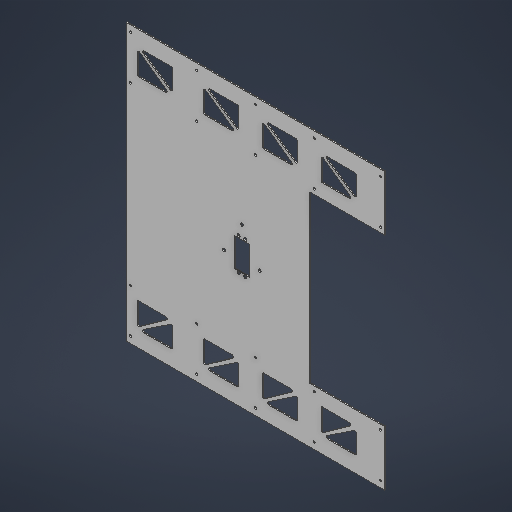
# Autodesk Inventor part: ВЕРХ 25-26
Saved by Autodesk Inventor 2026.2 (Build 302298000, 298)
## iProperties
Created: 2025-09-28
Part Number: ВЕРХ 25-26
Material: Типовые
Document SubType Name: Modeling
Designer: GameHD
Density: 1 g/cm^3
Appearance: По умолчанию
Author: GameHD
Autodesk Inventor part; units mm, degrees
(part 1 of 2)
ref_plane "YZ Plane" through (0, 0, 0) normal (1, 0, 0) x (0, 1, 0)
ref_plane "XZ Plane" through (0, 0, 0) normal (0, 1, 0) x (-1, 0, 0)
ref_plane "XY Plane" through (0, 0, 0) normal (0, 0, 1) x (1, 0, 0)
sketch "Эскиз1" plane through (0, 0, 0) normal (0, 0, 1) x (1, 0, 0)
  line L0 (0, 0) -> (380, 0)
  line L1 (380, 0) -> (380, 406)
  line L2 (380, 406) -> (0, 406)
  line L3 (0, 406) -> (0, 0)
  circle A0 centre (189.9999, 9.5) radius 1.625
  circle A1 centre (276.4236, 9.5) radius 1.625
  circle A2 centre (103.5763, 9.5) radius 1.625
  circle A3 centre (373.8998, 9.5) radius 1.625
  circle A4 centre (6.1, 9.5) radius 1.625
  line L4 (0, -31.725) -> (0, 41.275)
  line L5 (0, 203) -> (417.5125, 203)
  circle A5 centre (189.9999, 396.5) radius 1.625
  circle A6 centre (276.4236, 396.5) radius 1.625
  circle A7 centre (373.8998, 396.5) radius 1.625
  circle A8 centre (103.5763, 396.5) radius 1.625
  circle A9 centre (6.1, 396.5) radius 1.625
  circle A10 centre (189.9999, 73.9532) radius 1.625
  circle A11 centre (276.4236, 73.9532) radius 1.625
  circle A12 centre (373.8998, 73.9532) radius 1.625
  circle A13 centre (103.5763, 73.9532) radius 1.625
  circle A14 centre (6.1, 73.9532) radius 1.625
  circle A15 centre (189.9999, 332.0468) radius 1.625
  circle A16 centre (103.5763, 332.0468) radius 1.625
  circle A17 centre (373.8998, 332.0468) radius 1.625
  circle A18 centre (6.1, 332.0468) radius 1.625
  circle A19 centre (276.4236, 332.0468) radius 1.625
  line L6 (380, 203) -> (280, 203)
  line L7 (280, 203) -> (280, 81)
  line L8 (280, 81) -> (380, 81)
  line L9 (380, 81) -> (380, 203)
  line L10 (280, 203) -> (280, 325)
  line L11 (280, 325) -> (380, 325)
  circle A20 centre (6.1, 401.6) radius 1.625 projected
  arc A21 (257.5001, 384.25) -> (253.5001, 388.25) centre (253.5001, 384.25) ccw projected
  line L12 (253.5001, 388.25) -> (186.5001, 388.25) projected
  arc A22 (186.5001, 388.25) -> (182.5001, 384.25) centre (186.5001, 384.25) ccw projected
  line L13 (182.5001, 384.25) -> (182.5001, 342.25) projected
  arc A23 (182.5001, 342.25) -> (186.5001, 338.25) centre (186.5001, 342.25) ccw projected
  line L14 (186.5001, 338.25) -> (253.5001, 338.25) projected
  arc A24 (253.5001, 338.25) -> (257.5001, 342.25) centre (253.5001, 342.25) ccw projected
  line L15 (257.5001, 342.25) -> (257.5001, 384.25) projected
  line L16 (253.5001, 67.75) -> (186.5001, 67.75) projected
  arc A25 (186.5001, 67.75) -> (182.5001, 63.75) centre (186.5001, 63.75) ccw projected
  line L17 (182.5001, 63.75) -> (182.5001, 21.75) projected
  arc A26 (182.5001, 21.75) -> (186.5001, 17.75) centre (186.5001, 21.75) ccw projected
  line L18 (186.5001, 17.75) -> (253.5001, 17.75) projected
  arc A27 (253.5001, 17.75) -> (257.5001, 21.75) centre (253.5001, 21.75) ccw projected
  line L19 (257.5001, 21.75) -> (257.5001, 63.75) projected
  arc A28 (257.5001, 63.75) -> (253.5001, 67.75) centre (253.5001, 63.75) ccw projected
  arc A29 (148.6202, 331.9218) -> (145.3798, 331.9218) centre (147, 332.0468) ccw projected
  arc A30 (145.3798, 331.9218) -> (148.6202, 331.9218) centre (147, 331.7968) ccw projected
  arc A31 (371.3798, 314.6718) -> (374.6202, 314.6718) centre (373, 314.5468) ccw projected
  arc A32 (374.6202, 314.6718) -> (371.3798, 314.6718) centre (373, 314.7968) ccw projected
  arc A33 (231.3798, 74.0782) -> (234.6202, 74.0782) centre (233, 73.9532) ccw projected
  arc A34 (234.6202, 74.0782) -> (231.3798, 74.0782) centre (233, 74.2032) ccw projected
  arc A35 (5.38, 74.0782) -> (8.6204, 74.0782) centre (7.0002, 73.9532) ccw projected
  arc A36 (8.6204, 74.0782) -> (5.38, 74.0782) centre (7.0002, 74.2032) ccw projected
  arc A37 (148.6202, 91.3282) -> (145.3798, 91.3282) centre (147, 91.4532) ccw projected
  arc A38 (145.3798, 91.3282) -> (148.6202, 91.3282) centre (147, 91.2032) ccw projected
  arc A39 (374.6202, 91.3282) -> (371.3798, 91.3282) centre (373, 91.4532) ccw projected
  arc A40 (371.3798, 91.3282) -> (374.6202, 91.3282) centre (373, 91.2032) ccw projected
  arc A41 (231.3798, 314.6718) -> (234.6202, 314.6718) centre (233, 314.5468) ccw projected
  arc A42 (234.6202, 314.6718) -> (231.3798, 314.6718) centre (233, 314.7968) ccw projected
  arc A43 (5.38, 314.6718) -> (8.6204, 314.6718) centre (7.0002, 314.5468) ccw projected
  arc A44 (8.6204, 314.6718) -> (5.38, 314.6718) centre (7.0002, 314.7968) ccw projected
  arc A45 (145.3798, 314.6718) -> (148.6202, 314.6718) centre (147, 314.5468) ccw projected
  arc A46 (148.6202, 314.6718) -> (145.3798, 314.6718) centre (147, 314.7968) ccw projected
  arc A47 (374.6202, 331.9218) -> (371.3798, 331.9218) centre (373, 332.0468) ccw projected
  arc A48 (371.3798, 331.9218) -> (374.6202, 331.9218) centre (373, 331.7968) ccw projected
  arc A49 (234.6202, 91.3282) -> (231.3798, 91.3282) centre (233, 91.4532) ccw projected
  arc A50 (231.3798, 91.3282) -> (234.6202, 91.3282) centre (233, 91.2032) ccw projected
  arc A51 (8.6204, 91.3282) -> (5.38, 91.3282) centre (7.0002, 91.4532) ccw projected
  arc A52 (5.38, 91.3282) -> (8.6204, 91.3282) centre (7.0002, 91.2032) ccw projected
  arc A53 (145.3798, 74.0782) -> (148.6202, 74.0782) centre (147, 73.9532) ccw projected
  arc A54 (148.6202, 74.0782) -> (145.3798, 74.0782) centre (147, 74.2032) ccw projected
  arc A55 (371.3798, 74.0782) -> (374.6202, 74.0782) centre (373, 73.9532) ccw projected
  arc A56 (374.6202, 74.0782) -> (371.3798, 74.0782) centre (373, 74.2032) ccw projected
  arc A57 (234.6202, 331.9218) -> (231.3798, 331.9218) centre (233, 332.0468) ccw projected
  arc A58 (231.3798, 331.9218) -> (234.6202, 331.9218) centre (233, 331.7968) ccw projected
  arc A59 (8.6204, 331.9218) -> (5.38, 331.9218) centre (7.0002, 332.0468) ccw projected
  arc A60 (5.38, 331.9218) -> (8.6204, 331.9218) centre (7.0002, 331.7968) ccw projected
  circle A61 centre (373.9, 401.6) radius 1.625 projected
  circle A62 centre (374, 4.4) radius 1.625 projected
  circle A63 centre (6.1, 401.6) radius 1.625 projected
  circle A64 centre (6.1, 4.4) radius 1.625 projected
  circle A65 centre (190.0848, 396.5) radius 1.625 projected
  circle A66 centre (190.0848, 9.5) radius 1.625 projected
  circle A67 centre (233, 396.5) radius 1.625 projected
  circle A68 centre (233, 9.5) radius 1.625 projected
  circle A69 centre (134.0059, 201.175) radius 1.85 projected
  arc A70 (197.7028, 203) -> (198.309, 203) centre (198.0059, 201.175) ccw projected
  line L20 (198.309, 203) -> (197.7028, 203) projected
  circle A71 centre (134.0059, 142.375) radius 2 projected
  circle A72 centre (317.9941, 235.25) radius 2.1 projected
  circle A73 centre (62.0059, 170.75) radius 2.1 projected
  circle A74 centre (123.0059, 170.75) radius 2.1 projected
  circle A75 centre (317.9941, 170.75) radius 2.1 projected
  circle A76 centre (256.9941, 235.25) radius 2.1 projected
  circle A77 centre (62.0059, 235.25) radius 2.1 projected
  circle A78 centre (123.0059, 235.25) radius 2.1 projected
  circle A79 centre (256.9941, 170.75) radius 2.1 projected
  line L21 (49, 183) -> (13, 183) projected
  arc A80 (13, 183) -> (10, 180) centre (13, 180) ccw projected
  line L22 (10, 180) -> (10, 114) projected
  arc A81 (10, 114) -> (13, 111) centre (13, 114) ccw projected
  line L23 (13, 111) -> (49, 111) projected
  arc A82 (49, 111) -> (52, 114) centre (49, 114) ccw projected
  line L24 (52, 114) -> (52, 180) projected
  arc A83 (52, 180) -> (49, 183) centre (49, 180) ccw projected
  circle A84 centre (170.0002, 337.1128) radius 2.1 projected
  circle A85 centre (61.343, 305) radius 2.1 projected
  circle A86 centre (170.0002, 68.8872) radius 2.1 projected
  circle A87 centre (61.343, 191.9908) radius 2.1 projected
  circle A88 centre (65, 153.25) radius 2.1 projected
  circle A89 centre (65, 121) radius 2.1 projected
  arc A90 (32.152, 58) -> (34.152, 60) centre (32.152, 60) ccw projected
  line L25 (32.152, 58) -> (8, 58) projected
  arc A91 (8, 58) -> (5, 55) centre (8, 55) ccw projected
  line L26 (5, 55) -> (5, 11) projected
  arc A92 (5, 11) -> (8, 8) centre (8, 11) ccw projected
  line L27 (8, 8) -> (165, 8) projected
  arc A93 (165, 8) -> (168, 11) centre (165, 11) ccw projected
  line L28 (168, 11) -> (168, 55) projected
  arc A94 (168, 55) -> (165, 58) centre (165, 55) ccw projected
  line L29 (165, 58) -> (116.152, 58) projected
  arc A95 (114.152, 60) -> (116.152, 58) centre (116.152, 60) ccw projected
  line L30 (114.152, 60) -> (114.152, 72) projected
  arc A96 (114.152, 72) -> (112.152, 74) centre (112.152, 72) ccw projected
  line L31 (112.152, 74) -> (36.152, 74) projected
  arc A97 (36.152, 74) -> (34.152, 72) centre (36.152, 72) ccw projected
  line L32 (34.152, 72) -> (34.152, 60) projected
  arc A98 (345.848, 60) -> (347.848, 58) centre (347.848, 60) ccw projected
  line L33 (345.848, 60) -> (345.848, 72) projected
  arc A99 (345.848, 72) -> (343.848, 74) centre (343.848, 72) ccw projected
  line L34 (343.848, 74) -> (267.848, 74) projected
  arc A100 (267.848, 74) -> (265.848, 72) centre (267.848, 72) ccw projected
  line L35 (265.848, 72) -> (265.848, 10) projected
  arc A101 (265.848, 10) -> (267.848, 8) centre (267.848, 10) ccw projected
  line L36 (267.848, 8) -> (372, 8) projected
  arc A102 (372, 8) -> (375, 11) centre (372, 11) ccw projected
  line L37 (375, 11) -> (375, 55) projected
  arc A103 (375, 55) -> (372, 58) centre (372, 55) ccw projected
  line L38 (372, 58) -> (347.848, 58) projected
  arc A104 (347.848, 348) -> (345.848, 346) centre (347.848, 346) ccw projected
  line L39 (347.848, 348) -> (372, 348) projected
  arc A105 (372, 348) -> (375, 351) centre (372, 351) ccw projected
  line L40 (375, 351) -> (375, 395) projected
  arc A106 (375, 395) -> (372, 398) centre (372, 395) ccw projected
  line L41 (372, 398) -> (267.848, 398) projected
  arc A107 (267.848, 398) -> (265.848, 396) centre (267.848, 396) ccw projected
  line L42 (265.848, 396) -> (265.848, 334) projected
  arc A108 (265.848, 334) -> (267.848, 332) centre (267.848, 334) ccw projected
  line L43 (267.848, 332) -> (343.848, 332) projected
  arc A109 (343.848, 332) -> (345.848, 334) centre (343.848, 334) ccw projected
  line L44 (345.848, 334) -> (345.848, 346) projected
  arc A110 (34.152, 346) -> (32.152, 348) centre (32.152, 346) ccw projected
  line L45 (34.152, 346) -> (34.152, 334) projected
  arc A111 (34.152, 334) -> (36.152, 332) centre (36.152, 334) ccw projected
  line L46 (36.152, 332) -> (112.152, 332) projected
  arc A112 (112.152, 332) -> (114.152, 334) centre (112.152, 334) ccw projected
  line L47 (114.152, 334) -> (114.152, 346) projected
  arc A113 (116.152, 348) -> (114.152, 346) centre (116.152, 346) ccw projected
  line L48 (116.152, 348) -> (165, 348) projected
  arc A114 (165, 348) -> (168, 351) centre (165, 351) ccw projected
  line L49 (168, 351) -> (168, 395) projected
  arc A115 (168, 395) -> (165, 398) centre (165, 395) ccw projected
  line L50 (165, 398) -> (8, 398) projected
  arc A116 (8, 398) -> (5, 395) centre (8, 395) ccw projected
  line L51 (5, 395) -> (5, 351) projected
  arc A117 (5, 351) -> (8, 348) centre (8, 351) ccw projected
  line L52 (8, 348) -> (32.152, 348) projected
  line L53 (176.1539, 208.9063) -> (141.4028, 224.6949) projected
  arc A118 (141.4028, 224.6949) -> (137.8279, 220.0788) centre (140.1619, 221.9636) ccw projected
  line L54 (137.8279, 220.0788) -> (150.5778, 204.2902) projected
  arc A119 (150.5778, 204.2902) -> (152.9118, 203.175) centre (152.9118, 206.175) ccw projected
  line L55 (152.9118, 203.175) -> (174.913, 203.175) projected
  arc A120 (174.913, 203.175) -> (176.1539, 208.9063) centre (174.913, 206.175) ccw projected
  line L56 (164.9717, 173.5408) -> (165.9394, 174.4298) projected
  arc A121 (165.9394, 174.4298) -> (166.2437, 178.5238) centre (163.9097, 176.639) ccw projected
  line L57 (166.2437, 178.5238) -> (150.4677, 198.0598) projected
  arc A122 (150.4677, 198.0598) -> (148.1337, 199.175) centre (148.1337, 196.175) ccw projected
  line L58 (148.1337, 199.175) -> (145.4623, 199.175) projected
  arc A123 (145.4623, 199.175) -> (142.7128, 197.375) centre (145.4623, 196.175) ccw projected
  arc A124 (137.8059, 192.4681) -> (142.7128, 197.375) centre (134.0059, 201.175) ccw projected
  arc A125 (137.8059, 192.4681) -> (136.0059, 189.7186) centre (139.0059, 189.7186) ccw projected
  line L59 (136.0059, 189.7186) -> (136.0059, 175.75) projected
  arc A126 (136.0059, 175.75) -> (139.0059, 172.75) centre (139.0059, 175.75) ccw projected
  line L60 (139.0059, 172.75) -> (162.942, 172.75) projected
  arc A127 (162.942, 172.75) -> (164.9717, 173.5408) centre (162.942, 175.75) ccw projected
  line L61 (190.9762, 192.0005) -> (175.6931, 177.9592) projected
  arc A128 (175.6931, 177.9592) -> (177.7227, 172.75) centre (177.7227, 175.75) ccw projected
  line L62 (177.7227, 172.75) -> (193.0059, 172.75) projected
  arc A129 (193.0059, 172.75) -> (196.0059, 175.75) centre (193.0059, 175.75) ccw projected
  line L63 (196.0059, 175.75) -> (196.0059, 189.7914) projected
  arc A130 (196.0059, 189.7914) -> (190.9762, 192.0005) centre (193.0059, 189.7914) ccw projected
  line L64 (75.0034, 126.1924) -> (112.8628, 137.9196) projected
  arc A131 (112.8628, 137.9196) -> (112.4422, 143.7487) centre (111.9752, 140.7852) ccw projected
  line L65 (112.4422, 143.7487) -> (74.5828, 149.7151) projected
  arc A132 (74.5828, 149.7151) -> (71.1158, 146.7517) centre (74.1158, 146.7517) ccw projected
  line L66 (71.1158, 146.7517) -> (71.1158, 129.058) projected
  arc A133 (71.1158, 129.058) -> (75.0034, 126.1924) centre (74.1158, 129.058) ccw projected
  line L67 (273.1271, 237.25) -> (305.3345, 237.25) projected
  arc A134 (305.3345, 237.25) -> (307.3845, 242.4403) centre (305.3345, 240.25) ccw projected
  line L68 (307.3845, 242.4403) -> (293.7654, 255.1866) projected
  arc A135 (293.7654, 255.1866) -> (290.0188, 255.4704) centre (291.7154, 252.9963) ccw projected
  line L69 (290.0188, 255.4704) -> (271.4305, 242.7242) projected
  arc A136 (271.4305, 242.7242) -> (273.1271, 237.25) centre (273.1271, 240.25) ccw projected
  line L70 (237.7677, 178.4162) -> (207.2709, 194.1459) projected
  arc A137 (207.2709, 194.1459) -> (204.0022, 193.8065) centre (205.8957, 191.4797) ccw projected
  arc A138 (201.8059, 192.4681) -> (204.0022, 193.8065) centre (198.0059, 201.175) ccw projected
  arc A139 (201.8059, 192.4681) -> (200.0059, 189.7186) centre (203.0059, 189.7186) ccw projected
  line L71 (200.0059, 189.7186) -> (200.0059, 175.75) projected
  arc A140 (200.0059, 175.75) -> (203.0059, 172.75) centre (203.0059, 175.75) ccw projected
  line L72 (203.0059, 172.75) -> (236.3925, 172.75) projected
  arc A141 (236.3925, 172.75) -> (237.7677, 178.4162) centre (236.3925, 175.75) ccw projected
  line L73 (171.7502, 299.3659) -> (188.242, 287.4391) projected
  arc A142 (188.242, 287.4391) -> (191.758, 287.4391) centre (190, 289.8701) ccw projected
  line L74 (191.758, 287.4391) -> (215.7595, 304.7968) projected
  line L75 (215.7595, 304.7968) -> (173.5082, 304.7968) projected
  arc A143 (173.5082, 304.7968) -> (171.7502, 299.3659) centre (173.5082, 301.7968) ccw projected
  line L76 (265.3115, 243.3784) -> (285.9348, 257.5201) projected
  arc A144 (285.9348, 257.5201) -> (286.2882, 262.1846) centre (284.2382, 259.9942) ccw projected
  line L77 (286.2882, 262.1846) -> (245.2049, 300.6348) projected
  arc A145 (245.2049, 300.6348) -> (240.2828, 297.5781) centre (243.1549, 298.4444) ccw projected
  line L78 (240.2828, 297.5781) -> (255.6005, 246.7959) projected
  arc A146 (255.6005, 246.7959) -> (258.1178, 244.6833) centre (258.4726, 247.6622) ccw projected
  arc A147 (262.0259, 243.308) -> (258.1178, 244.6833) centre (256.9941, 235.25) ccw projected
  arc A148 (262.0259, 243.308) -> (265.3115, 243.3784) centre (263.6149, 245.8526) ccw projected
  arc A149 (72.6155, 242.4403) -> (74.6655, 237.25) centre (74.6655, 240.25) ccw projected
  line L79 (74.6655, 237.25) -> (111.9119, 237.25) projected
  arc A150 (111.9119, 237.25) -> (114.1595, 242.237) centre (111.9119, 240.25) ccw projected
  line L80 (114.1595, 242.237) -> (97.2953, 261.3129) projected
  arc A151 (97.2953, 261.3129) -> (92.9977, 261.5163) centre (95.0477, 259.3259) ccw projected
  line L81 (92.9977, 261.5163) -> (72.6155, 242.4403) projected
  line L82 (252.1574, 299.6064) -> (290.6344, 263.5955) projected
  arc A152 (290.6344, 263.5955) -> (294.3809, 263.3117) centre (292.6843, 265.7859) ccw projected
  line L83 (294.3809, 263.3117) -> (316.6907, 278.6098) projected
  arc A153 (316.6907, 278.6098) -> (317.9941, 281.084) centre (314.9941, 281.084) ccw projected
  line L84 (317.9941, 281.084) -> (317.9941, 301.7968) projected
  arc A154 (317.9941, 301.7968) -> (314.9941, 304.7968) centre (314.9941, 301.7968) ccw projected
  line L85 (314.9941, 304.7968) -> (254.2074, 304.7968) projected
  arc A155 (254.2074, 304.7968) -> (252.1574, 299.6064) centre (254.2074, 301.7968) ccw projected
  line L86 (196.7743, 281.2686) -> (212.8517, 269.6416) projected
  arc A156 (212.8517, 269.6416) -> (217.4768, 271.1895) centre (214.6097, 272.0726) ccw projected
  line L87 (217.4768, 271.1895) -> (226.6315, 300.9138) projected
  arc A157 (226.6315, 300.9138) -> (223.7644, 304.7968) centre (223.7644, 301.7968) ccw projected
  line L88 (223.7644, 304.7968) -> (223.5564, 304.7968) projected
  arc A158 (223.5564, 304.7968) -> (221.7984, 304.2277) centre (223.5564, 301.7968) ccw projected
  line L89 (221.7984, 304.2277) -> (196.7743, 286.1305) projected
  arc A159 (196.7743, 286.1305) -> (196.7743, 281.2686) centre (198.5323, 283.6996) ccw projected
  line L90 (209.1045, 197.7009) -> (247.729, 177.7791) projected
  arc A160 (247.729, 177.7791) -> (250.9978, 178.1185) centre (249.1042, 180.4453) ccw projected
  arc A161 (253.1941, 179.4569) -> (250.9978, 178.1185) centre (256.9941, 170.75) ccw projected
  arc A162 (253.1941, 179.4569) -> (254.9941, 182.2064) centre (251.9941, 182.2064) ccw projected
  line L91 (254.9941, 182.2064) -> (254.9941, 223.7936) projected
  arc A163 (254.9941, 223.7936) -> (253.1941, 226.5431) centre (251.9941, 223.7936) ccw projected
  arc A164 (251.3555, 227.6044) -> (253.1941, 226.5431) centre (256.9941, 235.25) ccw projected
  arc A165 (251.3555, 227.6044) -> (248.0743, 227.7877) centre (249.5749, 225.1899) ccw projected
  line L92 (248.0743, 227.7877) -> (208.9265, 205.1737) projected
  arc A166 (208.9265, 205.1737) -> (207.446, 202.2397) centre (210.4271, 202.576) ccw projected
  arc A167 (207.486, 200.561) -> (207.446, 202.2397) centre (198.0059, 201.175) ccw projected
  arc A168 (207.486, 200.561) -> (209.1045, 197.7009) centre (210.4797, 200.3671) ccw projected
  line L93 (290.6344, 142.4045) -> (250.0205, 104.3936) projected
  arc A169 (250.0205, 104.3936) -> (252.0705, 99.2032) centre (252.0705, 102.2032) ccw projected
  line L94 (252.0705, 99.2032) -> (314.9941, 99.2032) projected
  arc A170 (314.9941, 99.2032) -> (317.9941, 102.2032) centre (314.9941, 102.2032) ccw projected
  line L95 (317.9941, 102.2032) -> (317.9941, 124.916) projected
  arc A171 (317.9941, 124.916) -> (316.6907, 127.3902) centre (314.9941, 124.916) ccw projected
  line L96 (316.6907, 127.3902) -> (294.3809, 142.6883) projected
  arc A172 (294.3809, 142.6883) -> (290.6344, 142.4045) centre (292.6843, 140.2141) ccw projected
  line L97 (258.9941, 222.6864) -> (258.9941, 183.3136) projected
  arc A173 (258.9941, 183.3136) -> (264.1737, 181.2523) centre (261.9941, 183.3136) ccw projected
  line L98 (264.1737, 181.2523) -> (282.7918, 200.9386) projected
  arc A174 (282.7918, 200.9386) -> (282.7918, 205.0614) centre (280.6122, 203) ccw projected
  line L99 (282.7918, 205.0614) -> (264.1737, 224.7477) projected
  arc A175 (264.1737, 224.7477) -> (258.9941, 222.6864) centre (261.9941, 222.6864) ccw projected
  line L100 (73.6488, 153.9117) -> (89.4125, 151.4274) projected
  arc A176 (89.4125, 151.4274) -> (90.9794, 157.1819) centre (89.8795, 154.3908) ccw projected
  line L101 (90.9794, 157.1819) -> (75.2157, 163.3943) projected
  arc A177 (75.2157, 163.3943) -> (71.1158, 160.6033) centre (74.1158, 160.6033) ccw projected
  line L102 (71.1158, 160.6033) -> (71.1158, 156.8751) projected
  arc A178 (71.1158, 156.8751) -> (73.6488, 153.9117) centre (74.1158, 156.8751) ccw projected
  line L103 (136.0059, 165.75) -> (136.0059, 153.7586) projected
  arc A179 (136.0059, 153.7586) -> (141.0355, 151.5495) centre (139.0059, 153.7586) ccw projected
  line L104 (141.0355, 151.5495) -> (154.0874, 163.5408) projected
  arc A180 (154.0874, 163.5408) -> (152.0577, 168.75) centre (152.0577, 165.75) ccw projected
  line L105 (152.0577, 168.75) -> (139.0059, 168.75) projected
  arc A181 (139.0059, 168.75) -> (136.0059, 165.75) centre (139.0059, 165.75) ccw projected
  line L106 (187.6976, 229.0214) -> (194.3962, 214.0995) projected
  arc A182 (194.3962, 214.0995) -> (200.0002, 214.4451) centre (197.1331, 215.3281) ccw projected
  line L107 (200.0002, 214.4451) -> (204.5959, 229.367) projected
  arc A183 (204.5959, 229.367) -> (201.7288, 233.25) centre (201.7288, 230.25) ccw projected
  line L108 (201.7288, 233.25) -> (190.4345, 233.25) projected
  arc A184 (190.4345, 233.25) -> (187.6976, 229.0214) centre (190.4345, 230.25) ccw projected
  line L109 (96.148, 187.9448) -> (84.8346, 202.5382) projected
  arc A185 (84.8346, 202.5382) -> (80.7407, 203.156) centre (82.4637, 200.7001) ccw projected
  line L110 (80.7407, 203.156) -> (72.3928, 197.2996) projected
  arc A186 (72.3928, 197.2996) -> (71.1158, 194.8437) centre (74.1158, 194.8437) ccw projected
  line L111 (71.1158, 194.8437) -> (71.1158, 192.8793) projected
  arc A187 (71.1158, 192.8793) -> (73.1387, 190.0429) centre (74.1158, 192.8793) ccw projected
  line L112 (73.1387, 190.0429) -> (92.8, 183.2703) projected
  arc A188 (92.8, 183.2703) -> (96.148, 187.9448) centre (93.777, 186.1067) ccw projected
  line L113 (158.6531, 194.2902) -> (168.9546, 181.5336) projected
  arc A189 (168.9546, 181.5336) -> (173.3182, 181.2092) centre (171.2886, 183.4184) ccw projected
  line L114 (173.3182, 181.2092) -> (187.203, 193.9658) projected
  arc A190 (187.203, 193.9658) -> (185.1733, 199.175) centre (185.1733, 196.175) ccw projected
  line L115 (185.1733, 199.175) -> (160.9871, 199.175) projected
  arc A191 (160.9871, 199.175) -> (158.6531, 194.2902) centre (160.9871, 196.175) ccw projected
  line L116 (88.7233, 213.6423) -> (108.8956, 227.7941) projected
  arc A192 (108.8956, 227.7941) -> (107.1727, 233.25) centre (107.1727, 230.25) ccw projected
  line L117 (107.1727, 233.25) -> (74.1158, 233.25) projected
  arc A193 (74.1158, 233.25) -> (71.1158, 230.25) centre (74.1158, 230.25) ccw projected
  line L118 (71.1158, 230.25) -> (71.1158, 229.722) projected
  arc A194 (71.1158, 229.722) -> (71.9361, 227.6607) centre (74.1158, 229.722) ccw projected
  line L119 (71.9361, 227.6607) -> (84.8207, 214.0368) projected
  arc A195 (84.8207, 214.0368) -> (88.7233, 213.6423) centre (87.0003, 216.0982) ccw projected
  line L120 (138.452, 237.25) -> (174.984, 237.25) projected
  arc A196 (174.984, 237.25) -> (177.7209, 241.4786) centre (174.984, 240.25) ccw projected
  line L121 (177.7209, 241.4786) -> (168.7676, 261.4233) projected
  arc A197 (168.7676, 261.4233) -> (164.2727, 262.6256) centre (166.0307, 260.1947) ccw projected
  line L122 (164.2727, 262.6256) -> (136.694, 242.6809) projected
  arc A198 (136.694, 242.6809) -> (138.452, 237.25) centre (138.452, 240.25) ccw projected
  line L123 (183.2224, 163.8652) -> (190.6719, 154.6403) projected
  arc A199 (190.6719, 154.6403) -> (196.0059, 156.5251) centre (193.0059, 156.5251) ccw projected
  line L124 (196.0059, 156.5251) -> (196.0059, 165.75) projected
  arc A200 (196.0059, 165.75) -> (193.0059, 168.75) centre (193.0059, 165.75) ccw projected
  line L125 (193.0059, 168.75) -> (185.5564, 168.75) projected
  arc A201 (185.5564, 168.75) -> (183.2224, 163.8652) centre (185.5564, 165.75) ccw projected
  line L126 (104.4945, 108.7766) -> (129.3603, 99.741) projected
  arc A202 (129.3603, 99.741) -> (133.3849, 102.5606) centre (130.3849, 102.5606) ccw projected
  line L127 (133.3849, 102.5606) -> (133.3849, 108.9115) projected
  arc A203 (133.3849, 108.9115) -> (130.7069, 111.8942) centre (130.3849, 108.9115) ccw projected
  line L128 (130.7069, 111.8942) -> (105.8411, 114.5789) projected
  arc A204 (105.8411, 114.5789) -> (104.4945, 108.7766) centre (105.5191, 111.5962) ccw projected
  line L129 (266.425, 228.1886) -> (285.3145, 208.2154) projected
  arc A205 (285.3145, 208.2154) -> (289.6737, 208.2154) centre (287.4941, 210.2768) ccw projected
  line L130 (289.6737, 208.2154) -> (308.5632, 228.1886) projected
  arc A206 (308.5632, 228.1886) -> (306.3835, 233.25) centre (306.3835, 230.25) ccw projected
  line L131 (306.3835, 233.25) -> (268.6047, 233.25) projected
  arc A207 (268.6047, 233.25) -> (266.425, 228.1886) centre (268.6047, 230.25) ccw projected
  line L132 (76.1657, 251.2416) -> (90.4716, 264.6306) projected
  arc A208 (90.4716, 264.6306) -> (90.6693, 268.808) centre (88.4217, 266.821) ccw projected
  line L133 (90.6693, 268.808) -> (76.3634, 284.9901) projected
  arc A209 (76.3634, 284.9901) -> (71.1158, 283.0031) centre (74.1158, 283.0031) ccw projected
  line L134 (71.1158, 283.0031) -> (71.1158, 253.432) projected
  arc A210 (71.1158, 253.432) -> (76.1657, 251.2416) centre (74.1158, 253.432) ccw projected
  line L135 (133.824, 245.5418) -> (163.6065, 267.0802) projected
  arc A211 (163.6065, 267.0802) -> (164.5853, 270.7397) centre (161.8485, 269.5111) ccw projected
  line L136 (164.5853, 270.7397) -> (150.6579, 301.7648) projected
  arc A212 (150.6579, 301.7648) -> (145.0488, 301.4025) centre (147.921, 300.5362) ccw projected
  line L137 (145.0488, 301.4025) -> (129.1938, 248.8391) projected
  arc A213 (129.1938, 248.8391) -> (133.824, 245.5418) centre (132.066, 247.9727) ccw projected
  line L138 (71.8682, 296.1141) -> (93.4781, 271.6699) projected
  arc A214 (93.4781, 271.6699) -> (97.7757, 271.4666) centre (95.7258, 273.657) ccw projected
  line L139 (97.7757, 271.4666) -> (127.8426, 299.6064) projected
  arc A215 (127.8426, 299.6064) -> (125.7926, 304.7968) centre (125.7926, 301.7968) ccw projected
  line L140 (125.7926, 304.7968) -> (74.1158, 304.7968) projected
  arc A216 (74.1158, 304.7968) -> (71.1158, 301.7968) centre (74.1158, 301.7968) ccw projected
  line L141 (71.1158, 301.7968) -> (71.1158, 298.1011) projected
  arc A217 (71.1158, 298.1011) -> (71.8682, 296.1141) centre (74.1158, 298.1011) ccw projected
  line L142 (243.306, 242.6809) -> (221.8167, 258.2218) projected
  arc A218 (221.8167, 258.2218) -> (217.1916, 256.6739) centre (220.0587, 255.7909) ccw projected
  line L143 (217.1916, 256.6739) -> (212.4052, 241.133) projected
  arc A219 (212.4052, 241.133) -> (215.2723, 237.25) centre (215.2723, 240.25) ccw projected
  line L144 (215.2723, 237.25) -> (241.548, 237.25) projected
  arc A220 (241.548, 237.25) -> (243.306, 242.6809) centre (241.548, 240.25) ccw projected
  line L145 (207.6758, 239.367) -> (214.3683, 261.0966) projected
  arc A221 (214.3683, 261.0966) -> (213.2592, 264.4105) centre (211.5012, 261.9796) ccw projected
  line L146 (213.2592, 264.4105) -> (191.758, 279.96) projected
  arc A222 (191.758, 279.96) -> (188.242, 279.96) centre (190, 277.529) ccw projected
  line L147 (188.242, 279.96) -> (172.5476, 268.6099) projected
  arc A223 (172.5476, 268.6099) -> (171.5688, 264.9504) centre (174.3056, 266.179) ccw projected
  line L148 (171.5688, 264.9504) -> (183.2085, 239.0214) projected
  arc A224 (183.2085, 239.0214) -> (185.9454, 237.25) centre (185.9454, 240.25) ccw projected
  line L149 (185.9454, 237.25) -> (204.8087, 237.25) projected
  arc A225 (204.8087, 237.25) -> (207.6758, 239.367) centre (204.8087, 240.25) ccw projected
  line L150 (285.3145, 197.7846) -> (266.425, 177.8114) projected
  arc A226 (266.425, 177.8114) -> (268.6047, 172.75) centre (268.6047, 175.75) ccw projected
  line L151 (268.6047, 172.75) -> (306.3835, 172.75) projected
  arc A227 (306.3835, 172.75) -> (308.5632, 177.8114) centre (306.3835, 175.75) ccw projected
  line L152 (308.5632, 177.8114) -> (289.6737, 197.7846) projected
  arc A228 (289.6737, 197.7846) -> (285.3145, 197.7846) centre (287.4941, 195.7232) ccw projected
  line L153 (310.8145, 224.7477) -> (292.1964, 205.0614) projected
  arc A229 (292.1964, 205.0614) -> (292.1964, 200.9386) centre (294.376, 203) ccw projected
  line L154 (292.1964, 200.9386) -> (310.8145, 181.2523) projected
  arc A230 (310.8145, 181.2523) -> (315.9941, 183.3136) centre (312.9941, 183.3136) ccw projected
  line L155 (315.9941, 183.3136) -> (315.9941, 222.6864) projected
  arc A231 (315.9941, 222.6864) -> (310.8145, 224.7477) centre (312.9941, 222.6864) ccw projected
  line L156 (190.7609, 212.4306) -> (182.21, 231.4786) projected
  arc A232 (182.21, 231.4786) -> (179.4731, 233.25) centre (179.4731, 230.25) ccw projected
  line L157 (179.4731, 233.25) -> (146.0987, 233.25) projected
  arc A233 (146.0987, 233.25) -> (144.8578, 227.5187) centre (146.0987, 230.25) ccw projected
  line L158 (144.8578, 227.5187) -> (186.783, 208.4706) projected
  arc A234 (186.783, 208.4706) -> (190.7609, 212.4306) centre (188.024, 211.202) ccw projected
  line L159 (121.268, 155.5417) -> (111.9292, 167.5881) projected
  arc A235 (111.9292, 167.5881) -> (109.5582, 168.75) centre (109.5582, 165.75) ccw projected
  line L160 (109.5582, 168.75) -> (88.33, 168.75) projected
  arc A236 (88.33, 168.75) -> (87.2301, 162.9589) centre (88.33, 165.75) ccw projected
  line L161 (87.2301, 162.9589) -> (117.797, 150.9126) projected
  arc A237 (117.797, 150.9126) -> (121.268, 155.5417) centre (118.897, 153.7036) ccw projected
  line L162 (114.7758, 227.0332) -> (92.2222, 211.2108) projected
  arc A238 (92.2222, 211.2108) -> (91.7655, 206.6935) centre (93.9452, 208.7549) ccw projected
  line L163 (91.7655, 206.6935) -> (115.8263, 181.2523) projected
  arc A239 (115.8263, 181.2523) -> (121.0059, 183.3136) centre (118.0059, 183.3136) ccw projected
  line L164 (121.0059, 183.3136) -> (121.0059, 223.7936) projected
  arc A240 (121.0059, 223.7936) -> (119.2059, 226.5431) centre (118.0059, 223.7936) ccw projected
  arc A241 (118.0605, 227.1387) -> (119.2059, 226.5431) centre (123.0059, 235.25) ccw projected
  arc A242 (118.0605, 227.1387) -> (114.7758, 227.0332) centre (116.4988, 224.5773) ccw projected
  line L165 (285.9348, 148.4799) -> (283.4292, 150.1981) projected
  arc A243 (283.4292, 150.1981) -> (280.4301, 150.4264) centre (281.7326, 147.7239) ccw projected
  line L166 (280.4301, 150.4264) -> (242.0824, 131.9453) projected
  arc A244 (242.0824, 131.9453) -> (240.3849, 129.2428) centre (243.3849, 129.2428) ccw projected
  line L167 (240.3849, 129.2428) -> (240.3849, 107.7707) projected
  arc A245 (240.3849, 107.7707) -> (245.4348, 105.5804) centre (243.3849, 107.7707) ccw projected
  line L168 (245.4348, 105.5804) -> (286.2882, 143.8154) projected
  arc A246 (286.2882, 143.8154) -> (285.9348, 148.4799) centre (284.2382, 146.0058) ccw projected
  line L169 (139.3849, 123.75) -> (139.3849, 99.75) projected
  arc A247 (139.3849, 99.75) -> (142.3849, 96.75) centre (142.3849, 99.75) ccw projected
  line L170 (142.3849, 96.75) -> (231.3849, 96.75) projected
  arc A248 (231.3849, 96.75) -> (234.3849, 99.75) centre (231.3849, 99.75) ccw projected
  line L171 (234.3849, 99.75) -> (234.3849, 123.75) projected
  arc A249 (234.3849, 123.75) -> (231.3849, 126.75) centre (231.3849, 123.75) ccw projected
  line L172 (231.3849, 126.75) -> (142.3849, 126.75) projected
  arc A250 (142.3849, 126.75) -> (139.3849, 123.75) centre (142.3849, 123.75) ccw projected
  line L173 (134.7951, 300.6348) -> (100.3018, 268.3522) projected
  arc A251 (100.3018, 268.3522) -> (100.1042, 264.1749) centre (102.3518, 266.1619) ccw projected
  line L174 (100.1042, 264.1749) -> (116.9163, 245.1579) projected
  arc A252 (116.9163, 245.1579) -> (120.086, 244.2901) centre (119.1639, 247.1449) ccw projected
  arc A253 (121.8822, 244.6833) -> (120.086, 244.2901) centre (123.0059, 235.25) ccw projected
  arc A254 (121.8822, 244.6833) -> (124.3995, 246.7959) centre (121.5274, 247.6622) ccw projected
  line L175 (124.3995, 246.7959) -> (139.7172, 297.5781) projected
  arc A255 (139.7172, 297.5781) -> (134.7951, 300.6348) centre (136.8451, 298.4444) ccw projected
  arc A256 (133.3849, 129.2358) -> (133.1423, 131.1911) centre (125.3849, 129.2358) ccw projected
  arc A257 (133.1423, 131.1911) -> (131.1387, 133.318) centre (130.2332, 130.4579) ccw projected
  arc A258 (126.839, 136.1392) -> (131.1387, 133.318) centre (134.0059, 142.375) ccw projected
  arc A259 (126.839, 136.1392) -> (124.0903, 137.1304) centre (124.5758, 134.1699) ccw projected
  arc A260 (124.0903, 137.1304) -> (123.0178, 136.8776) centre (125.3849, 129.2358) ccw projected
  line L176 (123.0178, 136.8776) -> (88.6823, 126.242) projected
  arc A261 (88.6823, 126.242) -> (89.2479, 120.3937) centre (89.57, 123.3763) ccw projected
  line L177 (89.2479, 120.3937) -> (130.0629, 115.987) projected
  arc A262 (130.0629, 115.987) -> (133.3849, 118.9697) centre (130.3849, 118.9697) ccw projected
  line L178 (133.3849, 118.9697) -> (133.3849, 129.2358) projected
  line L179 (94.1155, 178.5864) -> (75.0928, 185.1391) projected
  arc A263 (75.0928, 185.1391) -> (71.1158, 182.3027) centre (74.1158, 182.3027) ccw projected
  line L180 (71.1158, 182.3027) -> (71.1158, 175.75) projected
  arc A264 (71.1158, 175.75) -> (74.1158, 172.75) centre (74.1158, 175.75) ccw projected
  line L181 (74.1158, 172.75) -> (93.1384, 172.75) projected
  arc A265 (93.1384, 172.75) -> (94.1155, 178.5864) centre (93.1384, 175.75) ccw projected
  line L182 (230.0831, 298.5311) -> (220.3001, 266.7669) projected
  arc A266 (220.3001, 266.7669) -> (221.4092, 263.4529) centre (223.1672, 265.8838) ccw projected
  line L183 (221.4092, 263.4529) -> (246.176, 245.5418) projected
  arc A267 (246.176, 245.5418) -> (250.8062, 248.8391) centre (247.934, 247.9727) ccw projected
  line L184 (250.8062, 248.8391) -> (235.8223, 298.5144) projected
  arc A268 (235.8223, 298.5144) -> (230.0831, 298.5311) centre (232.9502, 297.648) ccw projected
  arc A269 (189.299, 138.575) -> (189.9499, 137.34) centre (198.0059, 142.375) ccw projected
  arc A270 (189.299, 138.575) -> (186.5494, 140.375) centre (186.5494, 137.375) ccw projected
  line L185 (186.5494, 140.375) -> (150.91, 140.375) projected
  arc A271 (150.91, 140.375) -> (149.278, 134.8577) centre (150.91, 137.375) ccw projected
  line L186 (149.278, 134.8577) -> (151.7846, 133.2327) projected
  arc A272 (151.7846, 133.2327) -> (153.4165, 132.75) centre (153.4165, 135.75) ccw projected
  line L187 (153.4165, 132.75) -> (187.4059, 132.75) projected
  arc A273 (187.4059, 132.75) -> (189.9499, 137.34) centre (187.4059, 135.75) ccw projected
  arc A274 (206.0618, 137.34) -> (207.3536, 140.6807) centre (198.0059, 142.375) ccw projected
  arc A275 (206.0618, 137.34) -> (208.6058, 132.75) centre (208.6058, 135.75) ccw projected
  line L188 (208.6058, 132.75) -> (233.8536, 132.75) projected
  arc A276 (233.8536, 132.75) -> (235.156, 133.0475) centre (233.8536, 135.75) ccw projected
  line L189 (235.156, 133.0475) -> (273.5281, 151.5404) projected
  arc A277 (273.5281, 151.5404) -> (273.9223, 156.7171) centre (272.2257, 154.2429) ccw projected
  line L190 (273.9223, 156.7171) -> (273.3304, 157.1229) projected
  arc A278 (273.3304, 157.1229) -> (270.9434, 157.5682) centre (271.6338, 154.6487) ccw projected
  line L191 (270.9434, 157.5682) -> (209.6151, 143.0652) projected
  arc A279 (209.6151, 143.0652) -> (207.3536, 140.6807) centre (210.3055, 140.1457) ccw projected
  line L192 (189.2522, 150.0316) -> (175.037, 167.6348) projected
  arc A280 (175.037, 167.6348) -> (172.703, 168.75) centre (172.703, 165.75) ccw projected
  line L193 (172.703, 168.75) -> (165.6695, 168.75) projected
  line L194 (165.6695, 168.75) -> (144.8087, 149.5842) projected
  arc A281 (144.8087, 149.5842) -> (146.8384, 144.375) centre (146.8384, 147.375) ccw projected
  line L195 (146.8384, 144.375) -> (186.5494, 144.375) projected
  arc A282 (186.5494, 144.375) -> (189.299, 146.175) centre (186.5494, 147.375) ccw projected
  arc A283 (189.5792, 146.7616) -> (189.299, 146.175) centre (198.0059, 142.375) ccw projected
  arc A284 (189.5792, 146.7616) -> (189.2522, 150.0316) centre (186.9182, 148.1468) ccw projected
  line L196 (207.463, 149.1435) -> (236.3657, 163.0465) projected
  arc A285 (236.3657, 163.0465) -> (235.0652, 168.75) centre (235.0652, 165.75) ccw projected
  line L197 (235.0652, 168.75) -> (203.0059, 168.75) projected
  arc A286 (203.0059, 168.75) -> (200.0059, 165.75) centre (203.0059, 165.75) ccw projected
  line L198 (200.0059, 165.75) -> (200.0059, 153.8314) projected
  arc A287 (200.0059, 153.8314) -> (201.8059, 151.0819) centre (203.0059, 153.8314) ccw projected
  arc A288 (204.2049, 149.5737) -> (201.8059, 151.0819) centre (198.0059, 142.375) ccw projected
  arc A289 (204.2049, 149.5737) -> (207.463, 149.1435) centre (206.1625, 151.847) ccw projected
  line L199 (238.3424, 233.25) -> (212.1924, 233.25) projected
  arc A290 (212.1924, 233.25) -> (209.3253, 231.133) centre (212.1924, 230.25) ccw projected
  line L200 (209.3253, 231.133) -> (203.666, 212.7581) projected
  arc A291 (203.666, 212.7581) -> (208.0337, 209.2774) centre (206.5331, 211.8751) ccw projected
  line L201 (208.0337, 209.2774) -> (239.843, 227.6523) projected
  arc A292 (239.843, 227.6523) -> (238.3424, 233.25) centre (238.3424, 230.25) ccw projected
  circle A293 centre (198.0059, 142.375) radius 2 projected
  line L202 (317.9941, 247.3847) -> (317.9941, 268.9588) projected
  arc A294 (317.9941, 268.9588) -> (313.2975, 271.433) centre (314.9941, 268.9588) ccw projected
  line L203 (313.2975, 271.433) -> (298.465, 261.2621) projected
  arc A295 (298.465, 261.2621) -> (298.1116, 256.5975) centre (300.1615, 258.7879) ccw projected
  line L204 (298.1116, 256.5975) -> (310.9962, 244.5387) projected
  arc A296 (310.9962, 244.5387) -> (314.2337, 243.9741) centre (313.0462, 246.729) ccw projected
  arc A297 (315.7141, 244.4723) -> (314.2337, 243.9741) centre (317.9941, 235.25) ccw projected
  arc A298 (315.7141, 244.4723) -> (317.9941, 247.3847) centre (314.9941, 247.3847) ccw projected
  line L205 (317.9941, 137.0412) -> (317.9941, 158.6153) projected
  arc A299 (317.9941, 158.6153) -> (315.7141, 161.5277) centre (314.9941, 158.6153) ccw projected
  arc A300 (314.2337, 162.0259) -> (315.7141, 161.5277) centre (317.9941, 170.75) ccw projected
  arc A301 (314.2337, 162.0259) -> (310.9962, 161.4613) centre (313.0462, 159.271) ccw projected
  line L206 (310.9962, 161.4613) -> (298.1116, 149.4025) projected
  arc A302 (298.1116, 149.4025) -> (298.465, 144.7379) centre (300.1615, 147.2121) ccw projected
  line L207 (298.465, 144.7379) -> (313.2975, 134.567) projected
  arc A303 (313.2975, 134.567) -> (317.9941, 137.0412) centre (314.9941, 137.0412) ccw projected
  line L208 (156.48, 298.5625) -> (167.3865, 274.2669) projected
  arc A304 (167.3865, 274.2669) -> (171.8814, 273.0646) centre (170.1234, 275.4955) ccw projected
  line L209 (171.8814, 273.0646) -> (183.2257, 281.2686) projected
  arc A305 (183.2257, 281.2686) -> (183.2257, 286.1305) centre (181.4677, 283.6996) ccw projected
  line L210 (183.2257, 286.1305) -> (160.9749, 302.2221) projected
  arc A306 (160.9749, 302.2221) -> (156.48, 298.5625) centre (159.2169, 299.7912) ccw projected
  circle A307 centre (5, 170.75) radius 1.5 projected
  circle A308 centre (5, 129.058) radius 1.5 projected
  line L211 (53.391, 192.079) -> (54.8002, 192.4285) projected
  arc A309 (54.8002, 192.4285) -> (56.8024, 194.0842) centre (54.078, 195.3403) ccw projected
  arc A310 (56.9059, 194.2955) -> (56.8024, 194.0842) centre (61.343, 191.9908) ccw projected
  arc A311 (56.9059, 194.2955) -> (56.987, 196.8923) centre (54.2436, 195.6783) ccw projected
  line L212 (56.987, 196.8923) -> (50.1126, 212.4273) projected
  arc A312 (50.1126, 212.4273) -> (45.1248, 213.204) centre (47.3692, 211.2133) ccw projected
  line L213 (45.1248, 213.204) -> (30.7357, 196.9815) projected
  arc A313 (30.7357, 196.9815) -> (32.98, 191.9908) centre (32.98, 194.9908) ccw projected
  line L214 (32.98, 191.9908) -> (52.6688, 191.9908) projected
  arc A314 (52.6688, 191.9908) -> (53.391, 192.079) centre (52.6688, 194.9908) ccw projected
  line L215 (41.1301, 261.9232) -> (35.4572, 270.1271) projected
  arc A315 (35.4572, 270.1271) -> (30.2462, 267.2069) centre (32.9896, 268.4209) ccw projected
  line L216 (30.2462, 267.2069) -> (34.9665, 256.5398) projected
  arc A316 (34.9665, 256.5398) -> (40.508, 256.6716) centre (37.7099, 257.7538) ccw projected
  line L217 (40.508, 256.6716) -> (41.4606, 259.1348) projected
  arc A317 (41.4606, 259.1348) -> (41.1301, 261.9232) centre (38.6625, 260.217) ccw projected
  line L218 (53.7933, 279.934) -> (47.1014, 262.631) projected
  arc A318 (47.1014, 262.631) -> (47.432, 259.8426) centre (49.8995, 261.5489) ccw projected
  line L219 (47.432, 259.8426) -> (54.3838, 249.7892) projected
  arc A319 (54.3838, 249.7892) -> (59.8512, 251.524) centre (56.8513, 251.4955) ccw projected
  line L220 (59.8512, 251.524) -> (59.5912, 278.8804) projected
  arc A320 (59.5912, 278.8804) -> (53.7933, 279.934) centre (56.5913, 278.8519) ccw projected
  arc A321 (57.2156, 236.683) -> (57.078, 234.4037) centre (62.0059, 235.25) ccw projected
  arc A322 (57.2156, 236.683) -> (56.809, 239.249) centre (54.3415, 237.5428) ccw projected
  line L221 (56.809, 239.249) -> (48.0061, 251.9794) projected
  arc A323 (48.0061, 251.9794) -> (42.7406, 251.3552) centre (45.5386, 250.2731) ccw projected
  line L222 (42.7406, 251.3552) -> (40.6333, 245.9064) projected
  arc A324 (40.6333, 245.9064) -> (40.6879, 243.6103) centre (43.4313, 244.8243) ccw projected
  line L223 (40.6879, 243.6103) -> (47.4724, 228.2787) projected
  arc A325 (47.4724, 228.2787) -> (52.4601, 227.5019) centre (50.2158, 229.4926) ccw projected
  line L224 (52.4601, 227.5019) -> (56.3657, 231.9052) projected
  arc A326 (56.3657, 231.9052) -> (57.078, 234.4037) centre (54.1213, 233.8959) ccw projected
  line L225 (54.5556, 223.8364) -> (52.4205, 221.4292) projected
  arc A327 (52.4205, 221.4292) -> (51.9214, 218.2245) centre (54.6648, 219.4385) ccw projected
  line L226 (51.9214, 218.2245) -> (53.9494, 213.6416) projected
  arc A328 (53.9494, 213.6416) -> (59.6925, 214.8096) centre (56.6928, 214.8556) ccw projected
  line L227 (59.6925, 214.8096) -> (59.7996, 221.7997) projected
  arc A329 (59.7996, 221.7997) -> (54.5556, 223.8364) centre (56.7999, 221.8457) ccw projected
  line L228 (10.1793, 288.3503) -> (10.1793, 204.601) projected
  arc A330 (10.1793, 204.601) -> (10.6534, 202.9824) centre (13.1793, 204.601) ccw projected
  arc A331 (10.6534, 202.9824) -> (18.3688, 201.4013) centre (15.2808, 205.9478) ccw projected
  arc A332 (18.3688, 201.4013) -> (19.7331, 202.9544) centre (16.9351, 204.0365) ccw projected
  line L229 (19.7331, 202.9544) -> (35.408, 243.4847) projected
  arc A333 (35.408, 243.4847) -> (35.3534, 245.7808) centre (32.61, 244.5668) ccw projected
  line L230 (35.3534, 245.7808) -> (15.9197, 289.6976) projected
  arc A334 (15.9197, 289.6976) -> (10.1793, 288.3503) centre (13.1763, 288.4837) ccw projected
  line L231 (45.8214, 270.4106) -> (57.2251, 299.8968) projected
  arc A335 (57.2251, 299.8968) -> (57.0205, 302.4869) centre (54.427, 300.979) ccw projected
  arc A336 (56.9474, 302.6171) -> (57.0205, 302.4869) centre (61.343, 305) ccw projected
  arc A337 (56.9474, 302.6171) -> (54.8423, 304.1397) centre (54.31, 301.1873) ccw projected
  line L232 (54.8423, 304.1397) -> (50.3342, 304.9524) projected
  arc A338 (50.3342, 304.9524) -> (49.8019, 305) centre (49.8019, 302) ccw projected
  line L233 (49.8019, 305) -> (21.928, 305) projected
  arc A339 (21.928, 305) -> (19.4605, 300.2937) centre (21.928, 302) ccw projected
  line L234 (19.4605, 300.2937) -> (40.5559, 269.7865) projected
  arc A340 (40.5559, 269.7865) -> (45.8214, 270.4106) centre (43.0234, 271.4928) ccw projected
  line L235 (29.9169, 202.0864) -> (45.1645, 219.2768) projected
  arc A341 (45.1645, 219.2768) -> (45.6635, 222.4814) centre (42.9201, 221.2675) ccw projected
  line L236 (45.6635, 222.4814) -> (41.0748, 232.8514) projected
  arc A342 (41.0748, 232.8514) -> (35.5333, 232.7195) centre (38.3314, 231.6374) ccw projected
  line L237 (35.5333, 232.7195) -> (24.8746, 205.1593) projected
  arc A343 (24.8746, 205.1593) -> (29.9169, 202.0864) centre (27.6726, 204.0771) ccw projected
  arc A344 (417.7779, 398.9889) -> (413.2002, 406) centre (413.2002, 401) ccw projected
  line L238 (417.7779, 398.9889) -> (380, 313) projected
  arc A345 (377, 310) -> (380, 313) centre (377, 313) ccw projected
  line L239 (377, 310) -> (326.5966, 310) projected
  line L240 (326.5966, 310) -> (326.5966, 309) projected
  line L241 (326.5966, 309) -> (378, 309) projected
  arc A346 (380, 307) -> (378, 309) centre (378, 307) ccw projected
  line L242 (380, 307) -> (380, 99) projected
  arc A347 (378, 97) -> (380, 99) centre (378, 99) ccw projected
  line L243 (378, 97) -> (326.5966, 97) projected
  line L244 (326.5966, 97) -> (326.5966, 96) projected
  line L245 (326.5966, 96) -> (377, 96) projected
  arc A348 (380, 93) -> (377, 96) centre (377, 93) ccw projected
  line L246 (380, 93) -> (417.7779, 7.0111) projected
  arc A349 (413.2002, 0) -> (417.7779, 7.0111) centre (413.2002, 5) ccw projected
  line L247 (413.2002, 0) -> (3, 0) projected
  arc A350 (0, 3) -> (3, 0) centre (3, 3) ccw projected
  line L248 (0, 3) -> (0, 403) projected
  arc A351 (3, 406) -> (0, 403) centre (3, 403) ccw projected
  line L249 (3, 406) -> (413.2002, 406) projected
  point P0 (0, 364.725)
  point P1 (380, 325)
  dimension "d0" = 380
  dimension "d1" = 406
  dimension "d3" = 0
  dimension "d4" = 0
  dimension "d5" = 0
  dimension "d6" = 0
  dimension "d8" = 100
  dimension "d9" = 122
  dimension "d83" = 9.5
  dimension "d84" = 9.5
  dimension "d85" = 0
  dimension "d86" = 0
  dimension "d87" = 0
  dimension "d88" = 0
  dimension "d89" = 0
  constraints: 24 end point, 20 centre point, 13 symmetric about line, 4 parallel, 3 horizontal, 2 midpoint, 2 perpendicular, 1 point on line, 10 other
  measures "d0" distance of L2.end L1.end
  measures "d1" distance of L1.end L0.end
  measures "d3" vertical distance of A4.centre A2.centre
  measures "d4" vertical distance of A2.centre A0.centre
  measures "d5" vertical distance of A0.centre A1.centre
  measures "d6" vertical distance of A1.centre A3.centre
  measures "d8" distance of L8.end L7.end
  measures "d9" distance of L7.end L6.end
  measures "d83" distance from line of L2 A9.centre
  measures "d84" distance from line of L0 A3.centre
  measures "d85" vertical distance of A12.centre A55.centre
  measures "d86" vertical distance of A12.centre A11.centre
  measures "d87" vertical distance of A35.centre A14.centre
  measures "d88" vertical distance of A14.centre A13.centre
  measures "d89" vertical distance of A10.centre A13.centre
extrude "Выдавливание1" add sketch "Эскиз1" along normal blind 1.5 contours L3 A350 L0 | A350 L3 L5 A330 A331 A332 L229 A343 L235 L213 A313 L214 A314 L211 A309 A310 A311 L212 L110 A186 L111 A187 L112 A188 L109 A185 L163 A239 L164 A69 A70 A166 A167 A168 L90 A160 A161 A162 L91 L97 A173 L98 L7 L150 A226 L151 L166 A244 L167 A245 L168 L93 A169 L94 L8 L1 L0 | L3 A351 L2 L1 L11 L10 L85 A155 L82 L77 A145 L78 A146 A147 A148 L76 L69 A136 L67 L131 A207 L129 L99 A175 L97 L5 L91 A163 A164 A165 L92 A166 A69 L164 A240 A241 A242 L162 A238 L163 A185 L110 L212 A312 L213 L235 A341 L236 A342 L237 A343 L229 A333 L230 A334 L228 A330 | L3 L2 A351 | A330 L228 A334 L230 A333 L229 L5 | L5 L229 A332 A331 A330 | L94 A169 L93 L7 | A343 L237 A342 L236 A341 L235 L5 | L5 L235 A343 | L168 A245 L167 A244 L166 L7 | L213 A312 L212 L5 | L5 L212 A311 A310 A309 L211 A314 L214 A313 L213 | L151 A226 L150 L7 | L10 L82 A155 L85 | L7 L98 A173 L97 L5 | L5 L97 A175 L99 L10 | L110 A185 L5 | L5 A185 L109 A188 L112 A187 L111 A186 L110 | L10 L76 A148 A147 A146 L78 A145 L77 | L91 A162 A161 A160 L90 A168 A167 A166 L5 | L5 A166 L92 A165 A164 A163 L91 | L129 A207 L131 L10 | L163 A238 L162 A242 A241 A240 L164 L5 | L5 L164 A239 L163 | L10 L67 A136 L69 | A70 L5 | A69 L5 | L5 A69 | A0 A66 | A1 L36 A101 L35 A100 L34 A11 A99 L33 A98 L38 A103 L37 A102 A3 | A2 L27 A92 A4 L26 A91 L25 A90 L32 A97 L31 A13 A96 L30 A95 L29 A94 L28 A93 | A5 A65 | A6 L41 A106 A7 L40 A105 L39 A104 L44 A109 L43 A19 A108 L42 A107 | A8 L50 A115 L49 A114 L48 A113 L47 A112 L46 A16 A111 L45 A110 L52 A117 L51 A116 A9 | A12 A55 A56 | A14 A36 A35 | A17 A48 A47 | A18 A59 A60 | A20 | L15 A24 L14 A23 L13 A22 L12 A21 | A28 L19 A27 L18 A26 L17 A25 L16 | A30 A29 | A34 A33 | A38 A37 | A42 A41 | A44 A43 | A46 A45 | A50 A49 | A52 A51 | A54 A53 | A58 A57 | A61 | A62 | A64 | A67 | A68 | A71 | A73 | A74 | A76 | A77 | A78 | A79 | A83 L24 A82 L23 A81 L22 A80 L21 | A84 | A85 | A86 | A87 | A88 | A89 | A120 L55 A119 L54 A118 L53 | A127 L60 A126 L59 A125 A124 A123 L58 A122 L57 A121 L56 | A130 L63 A129 L62 A128 L61 | A133 L66 A132 L65 A131 L64 | A141 L72 A140 L71 A139 A138 A137 L70 | A143 L75 L74 A142 L73 | L81 A151 L80 A150 L79 A149 | A159 L89 A158 L88 A157 L87 A156 L86 | A178 L102 A177 L101 A176 L100 | A181 L105 A180 L104 A179 L103 | A184 L108 A183 L107 A182 L106 | A191 L115 A190 L114 A189 L113 | A195 L119 A194 L118 A193 L117 A192 L116 | A198 L122 A197 L121 A196 L120 | A201 L125 A200 L124 A199 L123 | A204 L128 A203 L127 A202 L126 | A210 L134 A209 L133 A208 L132 | A213 L137 A212 L136 A211 L135 | A217 L141 A216 L140 A215 L139 A214 L138 | A220 L144 A219 L143 A218 L142 | A225 L149 A224 L148 A223 L147 A222 L146 A221 L145 | A234 L158 A233 L157 A232 L156 | A237 L161 A236 L160 A235 L159 | A250 L172 A249 L171 A248 L170 A247 L169 | A255 L175 A254 A253 A252 L174 A251 L173 | L178 A262 L177 A261 L176 A260 A259 A258 A257 A256 | A265 L181 A264 L180 A263 L179 | A268 L184 A267 L183 A266 L182 | A269 A273 L187 A272 L186 A271 L185 A270 | A274 A279 L191 A278 L190 A277 L189 A276 L188 A275 | A284 A283 A282 L195 A281 L194 L193 A280 L192 | A289 A288 A287 L198 A286 L197 A285 L196 | A292 L201 A291 L200 A290 L199 | A293 | A306 L210 A305 L209 A304 L208 | A307 | A308 | A317 L217 A316 L216 A315 L215 | A320 L220 A319 L219 A318 L218 | A321 A326 L224 A325 L223 A324 L222 A323 L221 A322 | A329 L227 A328 L226 A327 L225 | A340 L234 A339 L233 A338 L232 A337 A336 A335 L231 picked at (191.6675, 9.3775) picked at (191.6675, 396.3775) picked at (371.7644, 74.623) picked at (8.2584, 74.5477) picked at (371.7644, 331.377) picked at (8.2584, 331.4523)